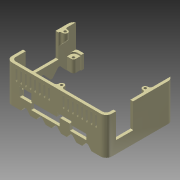
# Autodesk Inventor part: Caja SAV
Saved by Autodesk Inventor 2014 (Build 180170000, 170)
## iProperties
Created: 2014-09-10
Part Number: Caja SAV
Material: Nylon, molybdenum disulphide
Document SubType Name: Modeling
Designer: Rubén
Density: 1.13 g/cm^3
Appearance: Nylon 6
Mass: 39.8509 g
Surface Area: 258.502 cm^2
Volume: 35.2663 cm^3
Author: Rubén
Autodesk Inventor part; units mm, degrees
ref_plane "YZ Plane" through (0, 0, 0) normal (1, 0, 0) x (0, 1, 0)
ref_plane "XZ Plane" through (0, 0, 0) normal (0, 1, 0) x (-1, 0, 0)
ref_plane "XY Plane" through (0, 0, 0) normal (0, 0, 1) x (1, 0, 0)
sketch "Sketch1" plane through (0, 0, 0) normal (0, 1, 0) x (-1, 0, 0)
  line L0 (46.26, 32.385) -> (-46.26, 32.385) construction
  line L1 (-49.85, 28.795) -> (-49.85, -28.795) construction
  line L2 (-46.26, -32.385) -> (46.26, -32.385) construction
  line L3 (49.85, -28.795) -> (49.85, 28.795) construction
  arc A0 (-46.26, 32.385) -> (-49.85, 28.795) centre (-46.26, 28.795) ccw construction
  arc A1 (49.85, 28.795) -> (46.26, 32.385) centre (46.26, 28.795) ccw construction
  arc A2 (46.26, -32.385) -> (49.85, -28.795) centre (46.26, -28.795) ccw construction
  arc A3 (-49.85, -28.795) -> (-46.26, -32.385) centre (-46.26, -28.795) ccw construction
  line L4 (46.85, 33.385) -> (-46.85, 33.385)
  line L5 (-50.85, 29.385) -> (-50.85, -29.385)
  line L6 (-46.85, -33.385) -> (46.85, -33.385)
  line L7 (50.85, -29.385) -> (50.85, 29.385)
  line L8 (47.85, 36.385) -> (-47.85, 36.385)
  line L9 (-53.85, 30.385) -> (-53.85, -30.385)
  line L10 (-47.85, -36.385) -> (47.85, -36.385)
  line L11 (53.85, -30.385) -> (53.85, 30.385)
  arc A4 (50.85, 29.385) -> (46.85, 33.385) centre (46.85, 29.385) ccw
  arc A5 (46.85, -33.385) -> (50.85, -29.385) centre (46.85, -29.385) ccw
  arc A6 (-50.85, -29.385) -> (-46.85, -33.385) centre (-46.85, -29.385) ccw
  arc A7 (-46.85, 33.385) -> (-50.85, 29.385) centre (-46.85, 29.385) ccw
  arc A8 (-47.85, 36.385) -> (-53.85, 30.385) centre (-47.85, 30.385) ccw
  arc A9 (53.85, 30.385) -> (47.85, 36.385) centre (47.85, 30.385) ccw
  arc A10 (47.85, -36.385) -> (53.85, -30.385) centre (47.85, -30.385) ccw
  arc A11 (-53.85, -30.385) -> (-47.85, -36.385) centre (-47.85, -30.385) ccw
  point P0 (0, 0)
  point P1 (-49.85, -32.385)
  point P2 (-49.85, 32.385)
  point P3 (49.85, -32.385)
  point P4 (-50.85, -33.385)
  point P5 (-50.85, 33.385)
  point P6 (50.85, -33.385)
  point P7 (-53.85, -36.385)
  point P8 (-53.85, 36.385)
  point P9 (53.85, -36.385)
  dimension "d6" = 99.7
  dimension "d7" = 64.77
  dimension "d8" = 3.59
  dimension "d21" = 101.7
  dimension "d22" = 66.77
  dimension "d23" = 107.7
  dimension "d24" = 72.77
  dimension "d25" = 4
  dimension "d26" = 6
  dimension "d27" = 3
  dimension "d28" = 4
  dimension "d29" = 3
  dimension "d30" = 4
  dimension "d31" = 53.85
  dimension "d32" = 36.385
  constraints: 24 end point, 24 point on circle, 24 tangent, 18 point on line, 12 centre point, 9 equal radius, 6 parallel, 3 horizontal, 3 perpendicular
  measures "d6" distance of point (49.85, -32.385) point (-49.85, -32.385)
  measures "d7" distance of point (-49.85, -32.385) point (-49.85, 32.385)
  measures "d8" radius of A0
  measures "d21" distance of point (50.85, -33.385) point (-50.85, -33.385)
  measures "d22" distance of point (-50.85, -33.385) point (-50.85, 33.385)
  measures "d23" distance of point (53.85, -36.385) point (-53.85, -36.385)
  measures "d24" distance of point (-53.85, -36.385) point (-53.85, 36.385)
  measures "d25" radius of A4
  measures "d26" radius of A8
  measures "d27" distance between parallel lines of L11 L7
  measures "d28" distance between parallel lines of L11 L3
  measures "d29" distance between parallel lines of L4 L8
  measures "d30" distance between parallel lines of L0 L8
  measures "d31" distance from line of point (0, 0) L11
  measures "d32" distance from line of point (0, 0) L8
extrude "Extrusion1" add sketch "Sketch1" along normal blind 40
sketch "Sketch2" plane through (0, 0, 0) normal (0, 1, 0) x (-1, 0, 0)
  circle A0 centre (46.355, 28.575) radius 1.4
  circle A1 centre (-46.355, 28.575) radius 1.4
  circle A2 centre (46.355, -28.575) radius 1.4
  circle A3 centre (-46.355, -28.575) radius 1.4
  arc A4 (-46.355, 25.95) -> (-43.73, 28.575) centre (-46.355, 28.575) ccw
  line L0 (-46.355, 25.95) -> (-51.355, 25.95)
  arc A5 (43.73, 28.575) -> (46.355, 25.95) centre (46.355, 28.575) ccw
  arc A6 (46.355, -25.95) -> (43.73, -28.575) centre (46.355, -28.575) ccw
  arc A7 (-43.73, -28.575) -> (-46.355, -25.95) centre (-46.355, -28.575) ccw
  line L1 (-43.73, -28.575) -> (-43.73, -33.575)
  line L2 (-46.355, -25.95) -> (-51.355, -25.95)
  line L3 (-51.355, -25.95) -> (-51.355, -33.575)
  line L4 (-51.355, -33.575) -> (-43.73, -33.575)
  line L5 (46.355, -25.95) -> (51.355, -25.95)
  line L6 (43.73, -28.575) -> (43.73, -33.575)
  line L7 (43.73, -33.575) -> (51.355, -33.575)
  line L8 (51.355, -33.575) -> (51.355, -25.95)
  line L9 (46.355, 25.95) -> (51.355, 25.95)
  line L10 (43.73, 28.575) -> (43.73, 33.575)
  line L11 (43.73, 33.575) -> (51.355, 33.575)
  line L12 (51.355, 33.575) -> (51.355, 25.95)
  line L13 (-43.73, 28.575) -> (-43.73, 33.575)
  line L14 (-43.73, 33.575) -> (-51.355, 33.575)
  line L15 (-51.355, 33.575) -> (-51.355, 25.95)
  point P0 (0, 0)
  dimension "d2" = 2.8
  dimension "d3" = 2.8
  dimension "d4" = 2.8
  dimension "d5" = 2.8
  dimension "d9" = 28.575
  dimension "d12" = 57.15
  dimension "d13" = 92.71
  dimension "d16" = 54.4547
  dimension "d17" = 54.4547
  dimension "d18" = 54.4547
  dimension "d19" = 54.4547
  dimension "d20" = 57.15
  dimension "d35" = 5.25
  dimension "d36" = 5
  dimension "d39" = 5.25
  dimension "d40" = 5.25
  dimension "d41" = 5.25
  dimension "d42" = 5
  dimension "d43" = 5
  dimension "d44" = 5
  dimension "d45" = 5
  dimension "d46" = 5
  dimension "d47" = 5
  dimension "d48" = 5
  constraints: 32 end point, 9 tangent, 8 centre point, 8 perpendicular, 8 point on circle, 6 parallel, 4 coincident, 1 horizontal
  measures "d2" diameter of A1
  measures "d3" diameter of A0
  measures "d4" diameter of A2
  measures "d5" diameter of A3
  measures "d9" vertical distance of A0.centre point (0, 0)
  measures "d12" distance of A3.centre A1.centre
  measures "d13" distance of A3.centre A2.centre
  measures "d16" distance of A2.centre point (0, 0)
  measures "d17" distance of point (0, 0) A3.centre
  measures "d18" distance of A0.centre point (0, 0)
  measures "d19" distance of A1.centre point (0, 0)
  measures "d20" distance of A0.centre A2.centre
  measures "d35" diameter of A4
  measures "d36" distance of L0.start L0.end
  measures "d39" diameter of A5
  measures "d40" diameter of A6
  measures "d41" diameter of A7
  measures "d42" distance of L1.start L1.end
  measures "d43" distance of L2.start L2.end
  measures "d44" distance of L5.start L5.end
  measures "d45" distance of L6.start L6.end
  measures "d46" distance of L9.start L9.end
  measures "d47" distance of L10.start L10.end
  measures "d48" distance of L13.start L13.end
extrude "Extrusion2" add sketch "Sketch2" along normal blind 13
sketch "Sketch3" plane through (-47.85, 0, 36.385) normal (0, 0, 1) x (1, 0, 0)
  line L0 (95.7, 0) -> (0, 0) projected
  line L1 (95.7, 0) -> (95.7, 40) projected
  line L2 (0, 40) -> (95.7, 40) projected
  line L3 (0, 0) -> (0, 40) projected
  line L4 (47.85, 0) -> (47.85, 40) construction
  line L5 (0, 13) -> (95.7, 13) construction
  line L6 (0, 14.6) -> (95.7, 14.6) construction
  line L7 (8.85, 12) -> (20.21, 12)
  line L8 (8.85, 21.6) -> (20.55, 21.6)
  line L9 (8.35, 12.5) -> (8.35, 21.1)
  arc A0 (8.35, 12.5) -> (8.85, 12) centre (8.85, 12.5) ccw
  arc A1 (21.05, 21.1) -> (20.55, 21.6) centre (20.55, 21.1) ccw
  arc A2 (8.85, 21.6) -> (8.35, 21.1) centre (8.85, 21.1) ccw
  line L10 (64.16, 14) -> (64.16, 17.14)
  line L11 (61.9181, 14.1) -> (52.15, 14.1)
  line L12 (48.92, 14) -> (48.92, 17.14)
  line L13 (63.66, 17.64) -> (49.42, 17.64)
  arc A3 (49.42, 17.64) -> (48.92, 17.14) centre (49.42, 17.14) ccw
  arc A4 (64.16, 17.14) -> (63.66, 17.64) centre (63.66, 17.14) ccw
  line L14 (21.55, 13.5) -> (48.42, 13.5)
  line L15 (21.21, 6) -> (51.15, 6)
  line L16 (51.65, 13.6) -> (51.65, 6.5)
  arc A5 (20.71, 6.5) -> (21.21, 6) centre (21.21, 6.5) ccw
  arc A6 (51.15, 6) -> (51.65, 6.5) centre (51.15, 6.5) ccw
  line L17 (20.71, 6.5) -> (20.71, 11.5)
  line L18 (21.05, 21.1) -> (21.05, 14)
  arc A7 (20.71, 11.5) -> (20.21, 12) centre (20.21, 11.5) ccw
  arc A8 (21.05, 14) -> (21.55, 13.5) centre (21.55, 14) ccw
  arc A9 (48.42, 13.5) -> (48.92, 14) centre (48.42, 14) ccw
  arc A10 (52.15, 14.1) -> (51.65, 13.6) centre (52.15, 13.6) ccw
  line L19 (64.66, 13.5) -> (79.67, 13.5)
  line L20 (79.67, 7.5) -> (62.9181, 7.5)
  line L21 (62.4181, 13.6) -> (62.4181, 8)
  arc A11 (62.4181, 13.6) -> (61.9181, 14.1) centre (61.9181, 13.6) ccw
  arc A12 (64.16, 14) -> (64.66, 13.5) centre (64.66, 14) ccw
  arc A13 (62.4181, 8) -> (62.9181, 7.5) centre (62.9181, 8) ccw
  line L22 (49.3821, 4.1741) -> (52.8846, 0)
  line L23 (46.3179, 4.1741) -> (42.8154, 0)
  line L24 (42.8154, 0) -> (52.8846, 0)
  line L25 (65.8385, 4.1741) -> (69.341, 0)
  line L26 (62.7744, 4.1741) -> (59.2718, 0)
  line L27 (59.2718, 0) -> (69.341, 0)
  line L28 (32.9256, 4.1741) -> (36.4282, 0)
  line L29 (29.8615, 4.1741) -> (26.359, 0)
  line L30 (26.359, 0) -> (36.4282, 0)
  line L31 (16.4692, 4.1741) -> (19.9717, 0)
  line L32 (13.405, 4.1741) -> (9.9025, 0)
  line L33 (9.9025, 0) -> (19.9717, 0)
  line L34 (82.295, 4.1741) -> (85.7975, 0)
  line L35 (79.2308, 4.1741) -> (75.7283, 0)
  line L36 (75.7283, 0) -> (85.7975, 0)
  line L37 (90.79, 0) -> (90.79, 16.2211) construction
  line L38 (80.17, 8) -> (80.17, 13)
  arc A14 (80.17, 13) -> (79.67, 13.5) centre (79.67, 13) ccw
  arc A15 (79.67, 7.5) -> (80.17, 8) centre (79.67, 8) ccw
  line L39 (0, 24) -> (95.7, 24) construction
  line L40 (95.7, 37) -> (0, 37) construction
  line L41 (95.7, 37) -> (95.7, 24) construction
  line L42 (40, 37) -> (40, 24) construction
  line L43 (30, 37) -> (30, 24) construction
  line L44 (35, 37) -> (35, 24) construction
  line L45 (25, 37) -> (25, 24) construction
  line L46 (20, 37) -> (20, 24) construction
  line L47 (15, 37) -> (15, 24) construction
  line L48 (10, 37) -> (9.9025, 24) construction
  line L49 (5, 37) -> (5, 24) construction
  line L50 (90.7, 37) -> (90.7, 24) construction
  line L51 (85.7, 37) -> (85.7, 24) construction
  line L52 (80.7, 24) -> (80.7, 37) construction
  line L53 (75.7, 37) -> (75.7, 24) construction
  line L54 (70.7, 24) -> (70.7, 37) construction
  line L55 (65.7, 37) -> (65.7, 24) construction
  line L56 (60.7, 24) -> (60.7, 37) construction
  line L57 (55.7, 37) -> (55.7, 24) construction
  line L58 (5, 37) -> (5.9642, 35.8509)
  line L59 (5, 37) -> (6.5, 37) construction
  line L60 (5, 24) -> (5.9642, 25.1491)
  line L61 (5, 24) -> (6.5, 24) construction
  line L62 (5.9642, 25.1491) -> (5.9642, 35.8509)
  line L63 (5, 24) -> (4.0358, 25.1491)
  line L64 (5, 24) -> (6.5, 24) construction
  line L65 (4.0358, 25.1491) -> (4.0358, 35.8509)
  line L66 (4.0358, 35.8509) -> (5, 37)
  line L67 (10, 37) -> (10.9642, 35.8509)
  line L68 (10, 24) -> (10.9642, 25.1491)
  line L69 (10.9642, 25.1491) -> (10.9642, 35.8509)
  line L70 (10, 24) -> (9.0358, 25.1491)
  line L71 (9.0358, 25.1491) -> (9.0358, 35.8509)
  line L72 (9.0358, 35.8509) -> (10, 37)
  line L73 (15, 37) -> (15.9642, 35.8509)
  line L74 (15, 24) -> (15.9642, 25.1491)
  line L75 (15.9642, 25.1491) -> (15.9642, 35.8509)
  line L76 (15, 24) -> (14.0358, 25.1491)
  line L77 (14.0358, 25.1491) -> (14.0358, 35.8509)
  line L78 (14.0358, 35.8509) -> (15, 37)
  line L79 (20, 37) -> (20.9642, 35.8509)
  line L80 (20, 24) -> (20.9642, 25.1491)
  line L81 (20.9642, 25.1491) -> (20.9642, 35.8509)
  line L82 (20, 24) -> (19.0358, 25.1491)
  line L83 (19.0358, 25.1491) -> (19.0358, 35.8509)
  line L84 (19.0358, 35.8509) -> (20, 37)
  line L85 (25, 37) -> (25.9642, 35.8509)
  line L86 (25, 24) -> (25.9642, 25.1491)
  line L87 (25.9642, 25.1491) -> (25.9642, 35.8509)
  line L88 (25, 24) -> (24.0358, 25.1491)
  line L89 (24.0358, 25.1491) -> (24.0358, 35.8509)
  line L90 (24.0358, 35.8509) -> (25, 37)
  line L91 (30, 37) -> (30.9642, 35.8509)
  line L92 (30, 24) -> (30.9642, 25.1491)
  line L93 (30.9642, 25.1491) -> (30.9642, 35.8509)
  line L94 (30, 24) -> (29.0358, 25.1491)
  line L95 (29.0358, 25.1491) -> (29.0358, 35.8509)
  line L96 (29.0358, 35.8509) -> (30, 37)
  line L97 (35, 37) -> (35.9642, 35.8509)
  line L98 (35, 24) -> (35.9642, 25.1491)
  line L99 (35.9642, 25.1491) -> (35.9642, 35.8509)
  line L100 (35, 24) -> (34.0358, 25.1491)
  line L101 (34.0358, 25.1491) -> (34.0358, 35.8509)
  line L102 (34.0358, 35.8509) -> (35, 37)
  line L103 (40, 37) -> (40.9642, 35.8509)
  line L104 (40, 24) -> (40.9642, 25.1491)
  line L105 (40.9642, 25.1491) -> (40.9642, 35.8509)
  line L106 (40, 24) -> (39.0358, 25.1491)
  line L107 (39.0358, 25.1491) -> (39.0358, 35.8509)
  line L108 (39.0358, 35.8509) -> (40, 37)
  line L109 (55.7, 24) -> (56.6642, 25.1491)
  line L110 (56.6642, 25.1491) -> (56.6642, 35.8509)
  line L111 (54.7358, 25.1491) -> (54.7358, 35.8509)
  line L112 (55.7, 24) -> (54.7358, 25.1491)
  line L113 (54.7358, 35.8509) -> (55.7, 37)
  line L114 (55.7, 37) -> (56.6642, 35.8509)
  line L115 (60.7, 24) -> (59.7358, 25.1491)
  line L116 (59.7358, 25.1491) -> (59.7358, 35.8509)
  line L117 (59.7358, 35.8509) -> (60.7, 37)
  line L118 (60.7, 37) -> (61.6642, 35.8509)
  line L119 (61.6642, 25.1491) -> (61.6642, 35.8509)
  line L120 (60.7, 24) -> (61.6642, 25.1491)
  line L121 (65.7, 24) -> (64.7358, 25.1491)
  line L122 (64.7358, 25.1491) -> (64.7358, 35.8509)
  line L123 (64.7358, 35.8509) -> (65.7, 37)
  line L124 (65.7, 37) -> (66.6642, 35.8509)
  line L125 (66.6642, 25.1491) -> (66.6642, 35.8509)
  line L126 (65.7, 24) -> (66.6642, 25.1491)
  line L127 (70.7, 24) -> (69.7358, 25.1491)
  line L128 (69.7358, 25.1491) -> (69.7358, 35.8509)
  line L129 (69.7358, 35.8509) -> (70.7, 37)
  line L130 (70.7, 37) -> (71.6642, 35.8509)
  line L131 (71.6642, 25.1491) -> (71.6642, 35.8509)
  line L132 (70.7, 24) -> (71.6642, 25.1491)
  line L133 (75.7, 24) -> (74.7358, 25.1491)
  line L134 (74.7358, 25.1491) -> (74.7358, 35.8509)
  line L135 (74.7358, 35.8509) -> (75.7, 37)
  line L136 (75.7, 37) -> (76.6642, 35.8509)
  line L137 (76.6642, 25.1491) -> (76.6642, 35.8509)
  line L138 (75.7, 24) -> (76.6642, 25.1491)
  line L139 (80.7, 24) -> (79.7358, 25.1491)
  line L140 (79.7358, 25.1491) -> (79.7358, 35.8509)
  line L141 (79.7358, 35.8509) -> (80.7, 37)
  line L142 (80.7, 37) -> (81.6642, 35.8509)
  line L143 (81.6642, 25.1491) -> (81.6642, 35.8509)
  line L144 (80.7, 24) -> (81.6642, 25.1491)
  line L145 (85.7, 24) -> (84.7358, 25.1491)
  line L146 (84.7358, 25.1491) -> (84.7358, 35.8509)
  line L147 (84.7358, 35.8509) -> (85.7, 37)
  line L148 (85.7, 37) -> (86.6642, 35.8509)
  line L149 (86.6642, 25.1491) -> (86.6642, 35.8509)
  line L150 (85.7, 24) -> (86.6642, 25.1491)
  line L151 (90.7, 24) -> (89.7358, 25.1491)
  line L152 (89.7358, 25.1491) -> (89.7358, 35.8509)
  line L153 (89.7358, 35.8509) -> (90.7, 37)
  line L154 (90.7, 37) -> (91.6642, 35.8509)
  line L155 (91.6642, 25.1491) -> (91.6642, 35.8509)
  line L156 (90.7, 24) -> (91.6642, 25.1491)
  arc A16 (32.9256, 4.1741) -> (29.8615, 4.1741) centre (31.3936, 2.8886) ccw
  arc A17 (49.3821, 4.1741) -> (46.3179, 4.1741) centre (47.85, 2.8886) ccw
  arc A18 (65.8385, 4.1741) -> (62.7744, 4.1741) centre (64.3064, 2.8886) ccw
  arc A19 (82.295, 4.1741) -> (79.2308, 4.1741) centre (80.7629, 2.8886) ccw
  arc A20 (16.4692, 4.1741) -> (13.405, 4.1741) centre (14.9371, 2.8886) ccw
  point P0 (8.35, 12)
  point P1 (21.05, 0)
  point P2 (8.35, 21.6)
  point P3 (21.05, 21.6)
  point P4 (64.16, 14.1)
  point P5 (64.16, 17.64)
  point P6 (48.92, 17.64)
  point P7 (48.92, 13.4782)
  point P8 (51.65, 14.1)
  point P9 (62.4181, 14.1)
  point P10 (62.4181, 7.5)
  point P11 (90.79, 13.5)
  point P12 (80.17, 7.5)
  point P13 (47.85, 6)
  point P14 (64.3064, 6)
  point P15 (31.3936, 6)
  point P16 (14.9371, 6)
  point P17 (80.7629, 6)
  dimension "d53" = 17.64
  dimension "d55" = 13
  dimension "d56" = 21.6
  dimension "d57" = 64.16
  dimension "d58" = 48.92
  dimension "d60" = 8.35
  dimension "d61" = 14.6
  dimension "d62" = 74.65
  dimension "d88" = 0.5
  dimension "d91" = 0.5
  dimension "d92" = 0.5
  dimension "d93" = 21.05
  dimension "d94" = 7.5
  dimension "d96" = 33.2819
  dimension "d97" = 44.05
  dimension "d98" = 74.99
  dimension "d100" = 13.4782
  dimension "d101" = 74.65
  dimension "d107" = 90
  dimension "d108" = 90
  dimension "d109" = 90
  dimension "d123" = 6
  dimension "d124" = 50
  dimension "d125" = 9.9025
  dimension "d192" = 0.5
  dimension "d264" = 1.5
  dimension "d265" = 50
  dimension "d266" = 50
  dimension "d267" = 1.5
  dimension "d268" = 130
  dimension "d271" = 5
  dimension "d282" = 5
  dimension "d287" = 7.5
  dimension "d288" = 2
  constraints: 302 end point, 44 point on line, 44 tangent, 42 point on circle, 24 parallel, 21 centre point, 15 equal radius, 15 vertical, 10 perpendicular, 5 horizontal, 3 equal length, 2 collinear, 1 midpoint, 206 other
  measures "d53" distance between parallel lines of L0 L13
  measures "d55" distance between parallel lines of L0 L5
  measures "d56" distance between parallel lines of L0 L8
  measures "d57" distance between parallel lines of L3 L10
  measures "d58" distance between parallel lines of L3 L12
  measures "d60" distance between parallel lines of L3 L9
  measures "d61" distance between parallel lines of L6 L0
  measures "d62" distance from line of point (21.05, 0) L1
  measures "d88" radius of A9
  measures "d91" radius of A11
  measures "d92" radius of A0
  measures "d93" distance between parallel lines of L3 L18
  measures "d94" distance between parallel lines of L20 L0
  measures "d96" distance between parallel lines of L21 L1
  measures "d97" distance between parallel lines of L16 L1
  measures "d98" distance between parallel lines of L17 L1
  measures "d100" distance from line of point (48.92, 13.478) L0
  measures "d101" distance from line of point (21.05, 21.6) L1
  measures "d107" angle of L3 L27
  measures "d108" angle of L3 L30
  measures "d109" angle of L3 L33
  measures "d123" distance from line of L0 point (14.937, 6)
  measures "d124" angle of L0 L32
  measures "d125" distance of L32.end L0.end
  measures "d192" radius of A14
  measures "d264" distance of L49.start L58.end
  measures "d265" angle of L58 L59
  measures "d266" angle of L61 L60
  measures "d267" distance of L49.end L63.end
  measures "d268" angle of L64 L63
  measures "d271" distance of L49.end L68.start
  measures "d282" distance of L110.start L119.start
  measures "d287" distance between parallel lines of L15 L14
  measures "d288" radius of A16
extrude "Extrusion3" cut sketch "Sketch3" against normal blind 3 contours L0 L35 A19 L34 | L0 L26 A18 L25 | L32 A20 L31 L0 | L0 L23 A17 L22 | L29 A16 L28 L0 | A0 L9 A2 L8 A1 L18 A8 L14 A9 L12 A3 L13 A4 L10 A12 L19 A14 L38 A15 L20 A13 L21 A11 L11 A10 L16 A6 L15 A5 L17 A7 L7 | L58 L62 L60 L63 L65 L66 | L67 L69 L68 L70 L71 L72 | L73 L75 L74 L76 L77 L78 | L79 L81 L80 L82 L83 L84 | L85 L87 L86 L88 L89 L90 | L91 L93 L92 L94 L95 L96 | L97 L99 L98 L100 L101 L102 | L103 L105 L104 L106 L107 L108 | L112 L111 L113 L114 L110 L109 | L115 L116 L117 L118 L119 L120 | L121 L122 L123 L124 L125 L126 | L127 L128 L129 L130 L131 L132 | L133 L134 L135 L136 L137 L138 | L139 L140 L141 L142 L143 L144 | L145 L146 L147 L148 L149 L150 | L151 L152 L153 L154 L155 L156
sketch "Sketch5" plane through (-53.85, 0, -30.385) normal (-1, 0, 0) x (0, 0, 1)
  line L0 (60.77, 0) -> (60.77, 40) projected
  line L1 (0, 40) -> (60.77, 40) projected
  line L2 (0, 0) -> (0, 40) projected
  line L3 (0, 13) -> (60.77, 13) construction
  line L4 (48.285, 14.6) -> (14.185, 14.6) construction
  line L5 (30.385, 0) -> (30.385, 40) construction
  line L6 (13.685, 15.1) -> (13.685, 40)
  line L7 (48.785, 15.1) -> (48.785, 40)
  line L8 (14.185, 14.6) -> (48.285, 14.6)
  arc A0 (13.685, 15.1) -> (14.185, 14.6) centre (14.185, 15.1) ccw
  arc A1 (48.285, 14.6) -> (48.785, 15.1) centre (48.285, 15.1) ccw
  line L9 (31.8585, 7.6674) -> (38.2922, 0)
  line L10 (30.385, 9.4234) -> (40.3941, 9.4234) construction
  line L11 (28.845, 7.7255) -> (21.838, 0)
  line L12 (30.385, 9.4234) -> (40.8148, 9.4234) construction
  line L13 (21.838, 0) -> (38.2922, 0)
  line L14 (49.8816, 7.0428) -> (55.7912, 0)
  line L15 (46.8681, 7.1009) -> (40.4276, 0)
  line L16 (14.0816, 7.0428) -> (19.9912, 0)
  line L17 (11.0681, 7.1009) -> (4.6276, 0)
  arc A2 (14.0816, 7.0428) -> (11.0681, 7.1009) centre (12.5495, 5.7573) ccw
  arc A3 (31.8585, 7.6674) -> (28.845, 7.7255) centre (30.3264, 6.3818) ccw
  arc A4 (49.8816, 7.0428) -> (46.8681, 7.1009) centre (48.3495, 5.7573) ccw
  line L18 (4.6276, 0) -> (19.9912, 0)
  line L19 (40.4276, 0) -> (55.7912, 0)
  point P0 (48.4081, 8.7989)
  point P1 (55.6663, 0.1488)
  point P2 (40.5625, 0.1488)
  point P3 (12.6081, 8.7989)
  dimension "d134" = 50
  dimension "d144" = 11.985
  dimension "d145" = 47.085
  dimension "d289" = 2
  constraints: 34 end point, 13 point on line, 10 point on circle, 10 tangent, 5 centre point, 5 parallel, 3 equal radius, 3 perpendicular, 2 equal length, 2 horizontal, 1 collinear, 1 midpoint
  measures "d134" angle of L9 L10
  measures "d144" distance between parallel lines of L0 L7
  measures "d145" distance between parallel lines of L0 L6
  measures "d289" radius of A2
extrude "Extrusion4" cut sketch "Sketch5" against normal blind 3
sketch "Sketch6" plane through (53.85, 0, 30.385) normal (1, 0, 0) x (0, 0, -1)
  line L0 (60.77, 0) -> (60.77, 40) projected
  line L1 (0, 40) -> (60.77, 40) projected
  line L2 (0, 0) -> (0, 40) projected
  line L3 (30.385, 0) -> (30.385, 40) construction
  line L4 (5.185, 13) -> (60.77, 13) construction
  line L5 (60.77, 14.6) -> (0, 14.6) construction
  line L6 (5.185, 13) -> (22.485, 13)
  line L7 (22.985, 13.5) -> (22.985, 40)
  line L8 (4.685, 40) -> (4.685, 13.5)
  arc A0 (4.685, 13.5) -> (5.185, 13) centre (5.185, 13.5) ccw
  arc A1 (22.485, 13) -> (22.985, 13.5) centre (22.485, 13.5) ccw
  point P0 (0, 13)
  point P1 (22.985, 13)
  constraints: 12 end point, 10 point on line, 4 point on circle, 4 tangent, 2 centre point, 2 perpendicular, 1 midpoint
extrude "Extrusion5" cut sketch "Sketch6" against normal blind 3
sketch "Sketch7" plane through (47.85, 0, -36.385) normal (0, 0, -1) x (-1, 0, 0)
  line L0 (95.7, 0) -> (0, 0) projected
  line L1 (95.7, 0) -> (95.7, 40) projected
  line L2 (0, 40) -> (95.7, 40) projected
  line L3 (0, 0) -> (0, 40) projected
  line L4 (47.85, 0) -> (47.85, 40) construction
  line L5 (0, 13) -> (95.7, 13) construction
  line L6 (95.7, 14.6) -> (0, 14.6) construction
  line L7 (98.7, 40) -> (-3, 40)
  line L8 (47.85, 5) -> (54.377, 5) construction
  line L9 (47.85, 5) -> (54.377, 5) construction
  line L10 (64.306, 5) -> (70.833, 5) construction
  line L11 (64.306, 5) -> (70.833, 5) construction
  line L12 (-3, 14.6) -> (-3, 40)
  line L13 (98.7, 14.6) -> (98.7, 40)
  line L14 (5, 14.6) -> (5, 0)
  line L15 (90.7, 14.6) -> (90.7, 0)
  line L16 (-3, 14.6) -> (5, 14.6)
  line L17 (98.7, 14.6) -> (90.7, 14.6)
  line L18 (90.7, 0) -> (5, 0)
  dimension "d163" = 5
  dimension "d164" = 5
  dimension "d165" = 14.6
  dimension "d166" = 13
  dimension "d181" = 50.85
  dimension "d182" = 101.7
  constraints: 30 end point, 11 point on line, 4 horizontal, 4 perpendicular, 3 collinear, 2 parallel, 1 midpoint
  measures "d163" distance between parallel lines of L10 L0
  measures "d164" distance between parallel lines of L9 L0
  measures "d165" distance between parallel lines of L6 L0
  measures "d166" distance between parallel lines of L5 L0
  measures "d181" distance between parallel lines of L13 L4
  measures "d182" distance between parallel lines of L13 L12
extrude "Extrusion6" cut sketch "Sketch7" against normal blind 7 contours L0 L14 L16 L3 L2 L1 L17 L15 | L1 L7 L13 L17 | L3 L16 L12 L7
sketch "Sketch9" plane through (0, 40, 0) normal (0, 1, 0) x (1, 0, 0)
  line L0 (46.85, -33.385) -> (-46.85, -33.385) projected
  line L1 (-50.85, 16.7) -> (-50.85, 29.385) projected
  line L2 (43.5, 5.515) -> (-29, 5.515) construction
  line L3 (43.5, 26.115) -> (-29, 26.115) construction
  line L4 (-29, 5.515) -> (-29, 26.115) construction
  line L5 (43.5, 5.515) -> (43.5, 26.115) construction
  line L6 (7.25, 5.515) -> (7.25, 26.115) construction
  line L7 (-2.8, -30.885) -> (-2.8, -30.585)
  line L8 (0, -27.785) -> (0, -27.785)
  line L9 (2.8, -30.585) -> (2.8, -30.885)
  circle A0 centre (0, -30.585) radius 1.4
  arc A1 (0, -27.785) -> (-2.8, -30.585) centre (0, -30.585) ccw
  arc A2 (2.8, -30.585) -> (0, -27.785) centre (0, -30.585) ccw
  line L10 (-5.3, -33.385) -> (-5.3, -33.385)
  line L11 (5.3, -33.385) -> (5.3, -33.385)
  arc A3 (-5.3, -33.385) -> (-2.8, -30.885) centre (-5.3, -30.885) ccw
  arc A4 (2.8, -30.885) -> (5.3, -33.385) centre (5.3, -30.885) ccw
  line L12 (-5.3, -33.385) -> (5.3, -33.385)
  line L13 (-48.35, 18.5) -> (-48.05, 18.5)
  line L14 (-45.25, 21.3) -> (-45.25, 21.3)
  line L15 (-48.05, 24.1) -> (-48.35, 24.1)
  circle A5 centre (-48.05, 21.3) radius 1.4
  arc A6 (-45.25, 21.3) -> (-48.05, 24.1) centre (-48.05, 21.3) ccw
  arc A7 (-48.05, 18.5) -> (-45.25, 21.3) centre (-48.05, 21.3) ccw
  line L16 (50.85, 29.385) -> (50.85, -29.385) projected
  circle A8 centre (48.05, 11.5) radius 1.4
  line L17 (48.05, 8.7) -> (48.35, 8.7)
  line L18 (45.25, 11.5) -> (45.25, 11.5)
  line L19 (48.05, 14.3) -> (48.35, 14.3)
  line L20 (50.85, 16.8) -> (50.85, 16.8)
  line L21 (50.85, 6.2) -> (50.85, 6.2)
  arc A9 (48.05, 14.3) -> (45.25, 11.5) centre (48.05, 11.5) ccw
  arc A10 (45.25, 11.5) -> (48.05, 8.7) centre (48.05, 11.5) ccw
  arc A11 (48.35, 14.3) -> (50.85, 16.8) centre (48.35, 16.8) ccw
  arc A12 (50.85, 6.2) -> (48.35, 8.7) centre (48.35, 6.2) ccw
  line L22 (-53.85, 16.7) -> (-50.85, 16.7) projected
  line L23 (-48.35, 24.1) -> (-49.05, 24.1)
  line L24 (-48.35, 18.5) -> (-49.05, 18.5)
  line L25 (-50.85, 25.9) -> (-50.85, 25.9)
  line L26 (-50.85, 16.7) -> (-50.85, 16.7)
  arc A13 (-49.05, 18.5) -> (-50.85, 16.7) centre (-49.05, 16.7) ccw
  arc A14 (-50.85, 25.9) -> (-49.05, 24.1) centre (-49.05, 25.9) ccw
  line L27 (-50.85, 25.9) -> (-50.85, 16.7)
  point P0 (-50.85, -29.385)
  point P1 (-50.85, 35.5812)
  point P2 (0, 0)
  point P3 (-2.8, -27.785)
  point P4 (2.8, -27.785)
  point P5 (-2.8, -33.385)
  point P6 (2.8, -33.385)
  point P7 (-50.85, 18.5)
  point P8 (-45.25, 18.5)
  point P9 (-45.25, 24.1)
  point P10 (-50.85, 24.1)
  point P11 (50.85, 35.5812)
  point P12 (45.25, 8.7)
  point P13 (50.85, 8.7)
  point P14 (45.25, 14.3)
  point P15 (50.85, 14.3)
  point P16 (-50.85, -18.4)
  dimension "d212" = 2.5
  dimension "d213" = 2.5
  dimension "d214" = 2.5
  dimension "d225" = 5.6
  dimension "d226" = 5.6
  dimension "d229" = 2.8
  dimension "d231" = 2.8
  dimension "d239" = 2.8
  dimension "d240" = 5.6
  dimension "d241" = 2.5
  dimension "d242" = 2.5
  dimension "d243" = 2.8
  dimension "d244" = 2.5
  dimension "d253" = 1.8
  dimension "d254" = 1.8
  dimension "d255" = 1.8
  constraints: 48 end point, 34 point on line, 29 tangent, 25 point on circle, 15 centre point, 7 perpendicular, 6 equal radius, 4 horizontal, 3 parallel, 3 vertical, 2 midpoint, 1 collinear, 1 concentric, 5 other
  measures "d212" distance of point (-2.8, -33.385) L10.end
  measures "d213" distance of point (2.8, -33.385) L11.end
  measures "d214" radius of A3
  measures "d225" distance of point (-50.85, 18.5) point (-45.25, 18.5)
  measures "d226" distance of point (-45.25, 18.5) point (-45.25, 24.1)
  measures "d229" diameter of A5
  measures "d231" radius of A6
  measures "d239" diameter of A8
  measures "d240" distance of point (45.25, 8.7) point (45.25, 14.3)
  measures "d241" distance of point (50.85, 14.3) L20.end
  measures "d242" distance of point (50.85, 8.7) L21.end
  measures "d243" radius of A9
  measures "d244" radius of A11
  measures "d253" distance of point (-50.85, 24.1) L25.end
  measures "d254" distance of point (-50.85, 18.5) L22.end
  measures "d255" radius of A13
extrude "Extrusion7" add sketch "Sketch9" against normal blind 13
sketch "Sketch12" plane through (2.8, 40, 30.885) normal (1, 0, 0) x (0, 0, -1)
  line L0 (0, 0) -> (0, -13) projected
  line L1 (0.3, -13) -> (0, -13) projected
  line L2 (0.3, 0) -> (0.3, -13) projected
  line L3 (3.1, -13) -> (3.1, -6.3262)
  line L4 (-2.5, -13) -> (3.1, -6.3262)
  line L5 (3.1, -13) -> (-2.5, -13)
  point P0 (30.885, -40)
  dimension "d215" = 2.8
  dimension "d216" = 2.8
  dimension "d218" = 90
  dimension "d219" = 50
  dimension "d220" = 3.1
  constraints: 6 end point, 1 parallel
  measures "d215" distance of L1.start L4.start
  measures "d216" distance of L3.start L1.start
  measures "d218" angle of L2 L5
  measures "d219" angle of L1 L4
  measures "d220" distance between parallel lines of L0 L3
extrude "Extrusion9" cut sketch "Sketch12" along normal blind 2.5 and the other way blind 8.1
sketch "Sketch14" plane through (48.05, 40, -8.7) normal (0, 0, 1) x (1, 0, 0)
  line L0 (0.3, 0) -> (0, 0) projected
  line L1 (0.3, 0) -> (0.3, -13) projected
  line L2 (-2.8, -13) -> (-2.8, -6.3262)
  line L3 (-2.8, -13) -> (2.8, -13)
  line L4 (2.8, -13) -> (-2.8, -6.3262)
  point P0 (0, -13)
  point P1 (-48.05, -40)
  dimension "d245" = 2.8
  dimension "d246" = 5.6
  dimension "d247" = 50
  dimension "d248" = 13
  constraints: 6 end point, 1 parallel, 1 perpendicular
  measures "d245" distance of point (0, -13) L2.start
  measures "d246" distance of L2.start L3.end
  measures "d247" angle of L4 L3
  measures "d248" distance between parallel lines of L0 L3
extrude "Extrusion11" cut sketch "Sketch14" against normal blind 8.1 and the other way blind 2.5
sketch "Sketch15" plane through (-48.05, 40, -24.1) normal (0, 0, -1) x (-1, 0, 0)
  line L0 (2.8, -13) -> (-2.8, -6.3262)
  line L1 (-2.8, -6.3262) -> (-2.8, -13)
  line L2 (-2.8, -13) -> (2.8, -13)
  point P0 (0, -13)
  point P1 (-48.05, -40)
  dimension "d256" = 2.8
  dimension "d257" = 2.8
  constraints: 6 end point, 1 perpendicular
  measures "d256" distance of point (0, -13) L1.end
  measures "d257" distance of point (0, -13) L0.start
extrude "Extrusion12" cut sketch "Sketch15" along normal blind 1.8 and the other way blind 7.4
body "Solid1"
